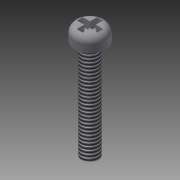
# Autodesk Inventor part: M2 Screw
Saved by Autodesk Inventor 2013 (Build 170138000, 138)
## iProperties
Created: 2012-10-31
Part Number: M2 Screw
Material: Generic
Document SubType Name: Modeling
Designer: uqgtayle
Density: 1 g/cm^3
Author: uqgtayle
Autodesk Inventor part; units mm, degrees
ref_plane "YZ Plane" through (0, 0, 0) normal (1, 0, 0) x (0, 1, 0)
ref_plane "XZ Plane" through (0, 0, 0) normal (0, 1, 0) x (-1, 0, 0)
ref_plane "XY Plane" through (0, 0, 0) normal (0, 0, 1) x (1, 0, 0)
sketch "Sketch1" plane through (0, 0, 0) normal (0, 0, 1) x (1, 0, 0)
  circle A0 centre (0, 0) radius 1
  dimension "d0" = 2
  constraints: 1 centre point, 1 coincident
  measures "d0" diameter of A0
extrude "Extrusion1" add sketch "Sketch1" along normal blind 12
thread "Thread1" size "M2x0.4" class "6g" standard "ANSI Metric M Profile" full length
sketch "Sketch2" plane through (0, 0, 12) normal (0, 0, 1) x (1, 0, 0)
  circle A0 centre (0, 0) radius 1 projected
  circle A1 centre (0, 0) radius 1.85
  dimension "d6" = 3.7
  constraints: 1 centre point, 1 coincident
  measures "d6" diameter of A1
extrude "Extrusion2" add sketch "Sketch2" along normal blind 1.7 contours A0 | A1
fillet "Fillet1" radius 0.8 1 edges at (-1.85, 0, 13.7)
sketch "Sketch3" plane through (0, 0, 13.7) normal (0, 0, 1) x (1, 0, 0)
  circle A0 centre (0, 0) radius 1.05 projected
  line L0 (-0.35, 1.25) -> (0.35, 1.25)
  line L1 (0.35, 1.25) -> (0.35, -1.25)
  line L2 (0.35, -1.25) -> (-0.35, -1.25)
  line L3 (-0.35, -1.25) -> (-0.35, 1.25)
  line L4 (-1.25, 0.35) -> (1.25, 0.35)
  line L5 (1.25, 0.35) -> (1.25, -0.35)
  line L6 (1.25, -0.35) -> (-1.25, -0.35)
  line L7 (-1.25, -0.35) -> (-1.25, 0.35)
  point P0 (0, 1.25)
  point P1 (0.35, 0)
  point P2 (-1.25, 0)
  point P3 (0, 0.35)
  dimension "d11" = 0.7
  dimension "d15" = 2.5
  dimension "d16" = 0.7
  dimension "d17" = 2.5
  constraints: 16 end point, 4 midpoint, 4 parallel, 2 horizontal, 2 horizontal alignment, 2 perpendicular, 2 vertical alignment
  measures "d11" distance of L1.end L2.end
  measures "d15" distance between parallel lines of L2 L0
  measures "d16" distance of L4.end L5.end
  measures "d17" distance of L4.start L4.end
extrude "Extrusion3" cut sketch "Sketch3" against normal blind 1 contours A0 L6 L1 L4 | A0 L4 L5 L6 | L1 L4 L3 A0 | A0 L3 L0 L1 | L1 L6 L3 L4 | L1 L2 L3 A0 | A0 L3 L6 L1 | L3 L6 A0 L4 | A0 L6 L7 L4
equation "\"d16\" = d11"
equation "\"d17\" = d15"
body "Solid1"
